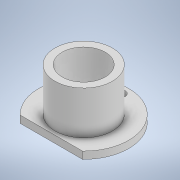
# Autodesk Inventor part: Buje de Resina
Saved by Autodesk Inventor 2020 (Build 240168000, 168)
## iProperties
Created: 2020-05-03
Part Number: Buje de Resina
Material: Acetal Resin, White
Document SubType Name: Modeling
Designer: Leon
Density: 1.425 g/cm^3
Appearance: Default
Mass: 2.35943 g
Surface Area: 19.2341 cm^2
Volume: 1.65574 cm^3
Author: Leon
Autodesk Inventor part; units mm, degrees
ref_plane "YZ Plane" through (0, 0, 0) normal (1, 0, 0) x (0, 1, 0)
ref_plane "XZ Plane" through (0, 0, 0) normal (0, 1, 0) x (-1, 0, 0)
ref_plane "XY Plane" through (0, 0, 0) normal (0, 0, 1) x (1, 0, 0)
ref_plane "Work Plane1" through (-12, 0, -11) normal (0, 0, 1) x (1, 0, 0)
sketch "Boceto6" plane through (0, 0, 0) normal (0, 1, 0) x (-1, 0, 0)
  circle A0 centre (9.21, 17.5305) radius 6
  circle A1 centre (9.21, 17.5305) radius 8
  arc A2 (0.5354, 26.5305) -> (17.8847, 26.5305) centre (9.21, 17.5305) ccw
  circle A3 centre (9.21, 7.5305) radius 1.5
  line L0 (9.21, 17.5305) -> (9.21, 26.5305)
  line L1 (9.21, 26.5305) -> (17.8847, 26.5305)
  line L2 (17.8847, 26.5305) -> (0.5354, 26.5305)
  point P0 (0, 0)
  dimension "d143" = 12
  dimension "d144" = 16
  dimension "d145" = 25
  dimension "d146" = 3
  dimension "d147" = 10
  dimension "d148" = 9
  constraints: 6 end point, 4 centre point, 2 coincident, 2 point on circle, 1 perpendicular, 1 vertical
  measures "d143" diameter of A0
  measures "d144" diameter of A1
  measures "d145" diameter of A2
  measures "d146" diameter of A3
  measures "d147" distance of A0.centre A3.centre
  measures "d148" distance of L0.start L0.end
extrude "Extrusión11" add sketch "Boceto6" along normal blind 12 contours A1
extrude "Extrusión12" add sketch "Boceto6" against normal blind 2 contours A1 | L2 L1 A2
